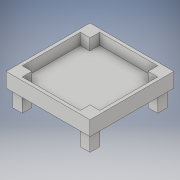
# Autodesk Inventor part: Pen
Saved by Autodesk Inventor 2017 (Build 210142000, 142)
## iProperties
Created: 2017-04-14
Part Number: Pen
Material: Generic
Document SubType Name: Modeling
Designer: Alex Tacescu
Density: 1 g/cm^3
Appearance: Default
Author: Alex Tacescu
Autodesk Inventor part; units mm, degrees
ref_plane "YZ Plane" through (0, 0, 0) normal (1, 0, 0) x (0, 1, 0)
ref_plane "XZ Plane" through (0, 0, 0) normal (0, 1, 0) x (-1, 0, 0)
ref_plane "XY Plane" through (0, 0, 0) normal (0, 0, 1) x (1, 0, 0)
sketch "Sketch1" plane through (0, 0, 0) normal (0, 1, 0) x (-1, 0, 0)
  line L0 (-152.4, 152.4) -> (152.4, 152.4) construction
  line L1 (152.4, 152.4) -> (152.4, -152.4) construction
  line L2 (152.4, -152.4) -> (-152.4, -152.4) construction
  line L3 (-152.4, -152.4) -> (-152.4, 152.4) construction
  line L4 (-152.4, 152.4) -> (152.4, -152.4) construction
  line L5 (152.4, 152.4) -> (-152.4, -152.4) construction
  line L6 (152.4, -152.4) -> (114.3, -152.4)
  line L7 (114.3, -152.4) -> (114.3, -114.3)
  line L8 (114.3, -114.3) -> (152.4, -114.3)
  line L9 (152.4, -114.3) -> (152.4, -152.4)
  line L10 (152.4, 152.4) -> (152.4, 114.3)
  line L11 (152.4, 114.3) -> (114.3, 114.3)
  line L12 (114.3, 114.3) -> (114.3, 152.4)
  line L13 (114.3, 152.4) -> (152.4, 152.4)
  line L14 (-152.4, 152.4) -> (-114.3, 152.4)
  line L15 (-114.3, 152.4) -> (-114.3, 114.3)
  line L16 (-114.3, 114.3) -> (-152.4, 114.3)
  line L17 (-152.4, 114.3) -> (-152.4, 152.4)
  line L18 (-152.4, -152.4) -> (-152.4, -114.3)
  line L19 (-152.4, -114.3) -> (-114.3, -114.3)
  line L20 (-114.3, -114.3) -> (-114.3, -152.4)
  line L21 (-114.3, -152.4) -> (-152.4, -152.4)
  point P0 (0, 0)
  dimension "d0" = 304.8
  dimension "d1" = 304.8
  dimension "d2" = 38.1
  dimension "d5" = 360
  constraints: 44 end point, 4 parallel, 2 horizontal, 2 midpoint, 2 perpendicular, 1 point on line, 33 other
  measures "d0" distance of L0.end L1.end
  measures "d1" distance of L1.end L2.end
  measures "d2" distance of L6.end L7.end
extrude "Extrusion1" add sketch "Sketch1" along normal blind 127
sketch "Sketch2" plane through (0, 127, 0) normal (0, 1, 0) x (1, 0, 0)
  line L0 (-114.3, 152.4) -> (-152.4, 152.4) projected
  line L1 (-152.4, 152.4) -> (-152.4, 114.3) projected
  line L2 (-152.4, 114.3) -> (-114.3, 114.3) projected
  line L3 (-114.3, 114.3) -> (-114.3, 152.4) projected
  line L4 (152.4, 114.3) -> (152.4, 152.4) projected
  line L5 (152.4, 152.4) -> (114.3, 152.4) projected
  line L6 (114.3, 152.4) -> (114.3, 114.3) projected
  line L7 (114.3, 114.3) -> (152.4, 114.3) projected
  line L8 (114.3, -152.4) -> (152.4, -152.4) projected
  line L9 (152.4, -152.4) -> (152.4, -114.3) projected
  line L10 (152.4, -114.3) -> (114.3, -114.3) projected
  line L11 (114.3, -114.3) -> (114.3, -152.4) projected
  line L12 (-152.4, -114.3) -> (-152.4, -152.4) projected
  line L13 (-152.4, -152.4) -> (-114.3, -152.4) projected
  line L14 (-114.3, -152.4) -> (-114.3, -114.3) projected
  line L15 (-114.3, -114.3) -> (-152.4, -114.3) projected
  line L16 (0, 231.14) -> (0, -231.14) projected
  line L17 (231.14, 0) -> (-231.14, 0) projected
  line L18 (-152.4, 152.4) -> (-152.4, -152.4)
  line L19 (-152.4, -152.4) -> (152.4, -152.4)
  line L20 (152.4, -152.4) -> (152.4, 152.4)
  line L21 (152.4, 152.4) -> (-152.4, 152.4)
  line L22 (-165.1, 165.1) -> (-165.1, -165.1)
  line L23 (-165.1, -165.1) -> (165.1, -165.1)
  line L24 (165.1, -165.1) -> (165.1, 165.1)
  line L25 (165.1, 165.1) -> (-165.1, 165.1)
  point P0 (0, 0)
  dimension "d9" = 12.7
  constraints: 16 end point, 3 collinear, 1 vertical, 3 other
  measures "d9" distance between parallel lines of L25 L21
extrude "Extrusion2" add sketch "Sketch2" against normal blind 57.15 contours L0 L1 L18 L17 L22 L25 L16 L21 | L16 L25 L24 L17 L20 L4 L5 L21 | L18 L12 L13 L19 L16 L23 L22 L17 | L19 L8 L9 L20 L17 L24 L23 L16
sketch "Sketch3" plane through (0, 69.85, 0) normal (0, -1, 0) x (1, 0, 0)
  line L0 (-165.1, 165.1) -> (165.1, 165.1) projected
  line L1 (-165.1, -165.1) -> (-165.1, 165.1) projected
  line L2 (-165.1, 165.1) -> (165.1, 165.1) projected
  line L3 (165.1, 165.1) -> (165.1, -165.1) projected
  line L4 (165.1, -165.1) -> (-165.1, -165.1) projected
  line L5 (114.3, 152.4) -> (-114.3, 152.4) projected
  line L6 (-114.3, 152.4) -> (-114.3, 114.3) projected
  line L7 (-114.3, 114.3) -> (-152.4, 114.3) projected
  line L8 (-152.4, 114.3) -> (-152.4, -114.3) projected
  line L9 (-152.4, -114.3) -> (-114.3, -114.3) projected
  line L10 (-114.3, -114.3) -> (-114.3, -152.4) projected
  line L11 (-114.3, -152.4) -> (114.3, -152.4) projected
  line L12 (114.3, -152.4) -> (114.3, -114.3) projected
  line L13 (114.3, -114.3) -> (152.4, -114.3) projected
  line L14 (152.4, -114.3) -> (152.4, 114.3) projected
  line L15 (152.4, 114.3) -> (114.3, 114.3) projected
  line L16 (114.3, 114.3) -> (114.3, 152.4) projected
  point P0 (0, 0)
extrude "Extrusion3" add sketch "Sketch3" against normal blind 12.7 contours L16 L15 L14 L13 L12 L11 L10 L9 L8 L7 L6 L5
chamfer "Chamfer1" distance 3.175 angle 45 16 edges at (-152.4, 0, 133.35) (-133.35, 0, 152.4) (-114.3, 0, 133.35) (-133.35, 0, 114.3) (-152.4, 0, -133.35) (-133.35, 0, -114.3) (-114.3, 0, -133.35) (-133.35, 0, -152.4) (114.3, 0, -133.35) (133.35, 0, -152.4) (133.35, 0, -114.3) (152.4, 0, -133.35) (133.35, 0, 114.3) (114.3, 0, 133.35) (133.35, 0, 152.4) (152.4, 0, 133.35)
body "Solid1"
